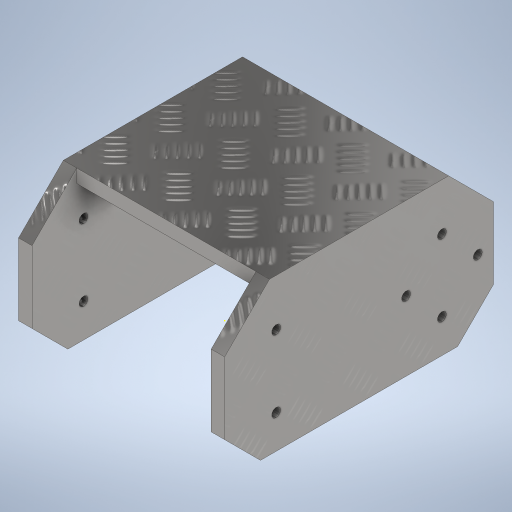
# Autodesk Inventor part: second_junction
Saved by Autodesk Inventor 2024 (Build 280153000, 153)
## iProperties
Created: 2024-02-16
Part Number: second_junction
Material: Generic
Document SubType Name: Modeling
Designer: kamil
Density: 1 g/cm^3
Appearance: Diamond Plate
Author: kamil
Autodesk Inventor part; units mm, degrees
ref_plane "YZ Plane" through (0, 0, 0) normal (1, 0, 0) x (0, 1, 0)
ref_plane "XZ Plane" through (0, 0, 0) normal (0, 1, 0) x (-1, 0, 0)
ref_plane "XY Plane" through (0, 0, 0) normal (0, 0, 1) x (1, 0, 0)
sketch "Sketch1" plane through (0, 0, 0) normal (0, 1, 0) x (-1, 0, 0)
  line L0 (0, 0) -> (46, 0)
  line L1 (46, 0) -> (46, -60)
  line L2 (46, -60) -> (0, -60)
  line L3 (0, -60) -> (0, 0)
  dimension "d0" = 46
  dimension "d1" = 60
  constraints: 8 end point, 2 parallel, 1 horizontal, 1 perpendicular
  measures "d0" distance of L1.end L2.end
  measures "d1" distance of L0.end L1.end
extrude "Extrusion1" add sketch "Sketch1" along normal blind 3
sketch "Sketch2" plane through (0, 0, 0) normal (0, -1, 0) x (1, 0, 0)
  line L0 (-46, -60) -> (-46, 0) projected
  line L1 (-46, 0) -> (0, 0) projected
  line L2 (-46, -60) -> (-43, -60)
  line L3 (-43, -60) -> (-43, 0)
  line L4 (-43, 0) -> (-46, 0)
  line L5 (-46, 0) -> (-46, -60)
  line L6 (0, -60) -> (-46, -60) projected
  line L7 (0, -60) -> (-3, -60)
  line L8 (-3, -60) -> (-3, 0)
  line L9 (-3, 0) -> (0, 0)
  line L10 (0, 0) -> (0, -60)
  dimension "d4" = 3
  dimension "d5" = 3
  dimension "d6" = 60
  constraints: 16 end point, 4 parallel, 2 horizontal, 2 perpendicular, 1 point on line
  measures "d4" distance of L4.end L3.end
  measures "d5" distance of L8.end L9.end
  measures "d6" distance of L7.end L8.end
extrude "Extrusion2" add sketch "Sketch2" along normal blind 31 contours L0 L1 L3 L2 | L8 L1 L10 L6
sketch "Sketch3" plane through (0, 3, 0) normal (1, 0, 0) x (0, 0, -1)
  line L0 (0, -3) -> (0, -34) projected
  line L1 (60, -3) -> (60, -34) projected
  line L2 (60, -18.5) -> (48.5, -18.5)
  circle A0 centre (40.5, -18.5) radius 1
  circle A1 centre (48.5, -26.5) radius 1
  circle A2 centre (56.5, -18.5) radius 1
  circle A3 centre (48.5, -10.5) radius 1
  line L3 (60, -34) -> (0, -34) projected
  dimension "d16" = 11.5
  dimension "d17" = 2
  dimension "d18" = 8
  dimension "d21" = 360
  dimension "d40" = 15.5
  constraints: 4 centre point, 2 end point, 1 midpoint, 9 other
  measures "d16" distance of L2.start L2.end
  measures "d17" diameter of A0
  measures "d18" distance of L2.end A0.centre
  measures "d40" distance from line of L3 L2.end
extrude "Extrusion3" cut sketch "Sketch3" against normal blind 3
sketch "Sketch4" plane through (0, 3, 0) normal (1, 0, 0) x (0, 0, -1)
  point P0 (0, -3)
sketch "Sketch5" plane through (0, 3, 0) normal (1, 0, 0) x (0, 0, -1)
  line L0 (0, -34) -> (0, 0) projected
  line L1 (0, -26) -> (8, -34)
  line L2 (60, -34) -> (0, -34) projected
  line L3 (52, -34) -> (60, -26)
  line L4 (60, 0) -> (60, -34) projected
  point P0 (0, -3)
  dimension "d25" = 8
  dimension "d26" = 8
  dimension "d27" = 8
  dimension "d28" = 8
  constraints: 4 end point, 4 point on line
  measures "d25" distance from line of L2 L1.start
  measures "d26" distance from line of L0 L1.end
  measures "d27" distance from line of L4 L3.start
  measures "d28" distance from line of L2 L3.end
extrude "Extrusion4" cut sketch "Sketch5" against normal blind 50
sketch "Sketch6" plane through (0, 3, 0) normal (0, 1, 0) x (1, 0, 0)
  line L0 (-3, 60) -> (-3, 0) projected
  line L1 (-43, 60) -> (-3, 60)
  line L2 (-3, 60) -> (-3, 50)
  line L3 (-3, 50) -> (-43, 50)
  line L4 (-43, 50) -> (-43, 60)
  line L5 (-43, 0) -> (-3, 0) projected
  line L6 (-3, 0) -> (-43, 0)
  line L7 (-43, 0) -> (-43, 10)
  line L8 (-43, 10) -> (-3, 10)
  line L9 (-3, 10) -> (-3, 0)
  point P0 (0, 0)
  dimension "d31" = 10
  dimension "d32" = 40
  dimension "d33" = 10
  constraints: 16 end point, 4 parallel, 2 horizontal, 2 perpendicular, 1 point on line
  measures "d31" distance of L1.end L2.end
  measures "d32" distance of L7.end L8.end
  measures "d33" distance of L6.end L7.end
extrude "Extrusion5" cut sketch "Sketch6" against normal blind 10
sketch "Sketch8" plane through (-46, 3, -60) normal (-1, 0, 0) x (0, 0, 1)
  line L0 (8, -34) -> (52, -34) projected
  line L1 (11.5, -34) -> (11.5, -18.5)
  line L2 (11.5, -34) -> (27, -34) construction
  circle A0 centre (11.5, -18.5) radius 1.25
  line L3 (0, -26) -> (0, 0) projected
  point P0 (60, -3)
  dimension "d38" = 15.5
  dimension "d39" = 90
  dimension "d41" = 2.5
  dimension "d42" = 11.5
  constraints: 4 end point, 2 perpendicular, 1 centre point, 1 coincident, 1 horizontal, 1 point on line
  measures "d38" distance of L1.start L1.end
  measures "d39" angle of L2 L1
  measures "d41" diameter of A0
  measures "d42" distance from line of L3 L1.end
extrude "Extrusion7" cut sketch "Sketch8" against normal blind 3
sketch "Sketch9" plane through (0, 3, 0) normal (1, 0, 0) x (0, 0, -1)
  line L0 (0, -26) -> (0, 0) projected
  line L1 (0, -18.5) -> (11.5, -18.5)
  line L2 (0, -18.5) -> (11.5, -18.5) construction
  line L3 (52, -34) -> (8, -34) projected
  circle A0 centre (11.5, -10.5) radius 1
  circle A1 centre (11.5, -26.5) radius 1
  point P0 (0, -3)
  dimension "d47" = 11.5
  dimension "d49" = 15.5
  dimension "d50" = 2
  dimension "d51" = 8
  constraints: 4 end point, 2 centre point, 1 collinear, 1 horizontal, 1 perpendicular, 1 point on line, 1 symmetric about line, 1 other
  measures "d47" distance of L1.start L1.end
  measures "d49" distance between parallel lines of L3 L1
  measures "d50" diameter of A0
  measures "d51" distance of L1.end A0.centre
extrude "Extrusion8" cut sketch "Sketch9" against normal blind 50
sketch "Sketch10" plane through (-46, 3, -60) normal (-1, 0, 0) x (0, 0, 1)
  line L0 (10, 0) -> (10, -3) projected
  line L1 (10, 0) -> (0, -10)
  line L2 (0, 0) -> (0, -26) projected
  line L3 (0, 0) -> (60, 0) projected
  line L4 (50, 0) -> (60, -10)
  line L5 (60, -26) -> (60, 0) projected
  point P0 (60, -3)
  dimension "d54" = 10
  dimension "d55" = 10
  dimension "d56" = 10
  dimension "d57" = 10
  constraints: 4 end point, 3 point on line
  measures "d54" distance from line of L2 L0.start
  measures "d55" distance from line of L3 L1.end
  measures "d56" distance from line of L5 L4.start
  measures "d57" distance from line of L3 L4.end
extrude "Extrusion9" cut sketch "Sketch10" against normal blind 50
body "Solid1"
